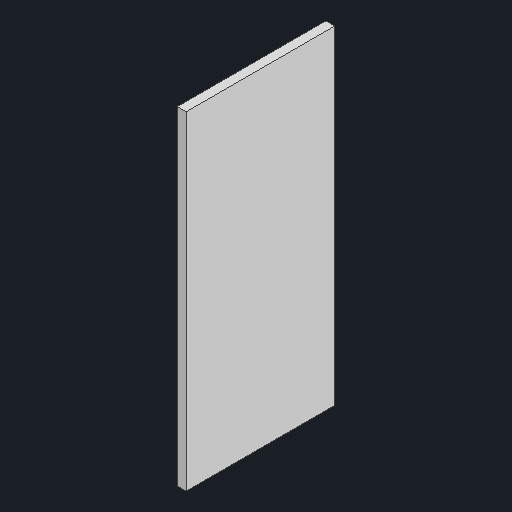
# Autodesk Inventor part: Sliding Plate
Saved by Autodesk Inventor 2022 (Build 260153000, 153)
## iProperties
Created: 2021-06-04
Part Number: Sliding Plate
Material: Generic
Document SubType Name: Modeling
Designer: saatvik123
Density: 1 g/cm^3
Appearance: Default
Author: saatvik123
## iProperties of the stored document Sliding Plate_3DPrint.ipt
Created: 2021-06-06
Part Number: Sliding Plate_3DPrint
Material: Generic
Document SubType Name: Modeling
Designer: sidsa
Density: 1 g/cm^3
Appearance: Default
Author: sidsa
Autodesk Inventor part; units mm, degrees
ref_plane "YZ Plane" through (0, 0, 0) normal (1, 0, 0) x (0, 1, 0)
ref_plane "XZ Plane" through (0, 0, 0) normal (0, 1, 0) x (-1, 0, 0)
ref_plane "XY Plane" through (0, 0, 0) normal (0, 0, 1) x (1, 0, 0)
sketch "Sketch1" plane through (0, 0, 0) normal (0, 0, 1) x (1, 0, 0)
  line L0 (16.256, -19.05) -> (16.256, -28.575) projected
  line L1 (18.796, -28.575) -> (16.256, -28.575) projected
  line L2 (18.796, -28.575) -> (18.796, -26.035) projected
  line L3 (18.796, -26.035) -> (21.336, -26.035) projected
  line L4 (25.4, 28.575) -> (25.4, -28.575) projected
  line L5 (21.336, 26.035) -> (18.796, 26.035) projected
  line L6 (18.796, 26.035) -> (18.796, 28.575) projected
  line L7 (16.256, 28.575) -> (18.796, 28.575) projected
  line L8 (16.256, 28.575) -> (16.256, 19.05) projected
  line L9 (21.336, 28.575) -> (25.4, 28.575) projected
  line L10 (-25.4, -19.05) -> (-25.4, 19.05) projected
  line L11 (25.4, -28.575) -> (21.336, -28.575) projected
  line L12 (16.256, -28.575) -> (18.796, -28.575)
  line L13 (18.796, -28.575) -> (18.796, 28.575)
  line L14 (18.796, 28.575) -> (16.256, 28.575)
  line L15 (16.256, 28.575) -> (16.256, -28.575)
  line L16 (16.764, -28.067) -> (18.288, -28.067)
  line L17 (18.288, -28.067) -> (18.288, 28.067)
  line L18 (18.288, 28.067) -> (16.764, 28.067)
  line L19 (16.764, 28.067) -> (16.764, -28.067)
  line L20 (21.336, -26.035) -> (21.336, -28.575) projected
  line L21 (21.336, 28.575) -> (21.336, 26.035) projected
  line L22 (16.256, 19.05) -> (-25.4, 19.05) projected
  line L23 (-25.4, -19.05) -> (16.256, -19.05) projected
  point P0 (0, 0)
  dimension "d0" = 0.508
  constraints: 16 end point, 4 parallel, 2 perpendicular, 1 horizontal, 3 other
  measures "d0" distance between parallel lines of L15 L19
extrude "Extrusion1" add sketch "Sketch1" along normal blind 25.4 contours L19 L18 L17 L16
body "Solid1"
